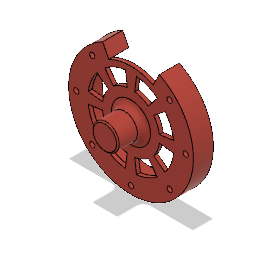
Hip Axis (Autodesk Fusion 360 design; units mm, degrees)
Autodesk Fusion 360 part; units mm, degrees
sketch "base" plane through (0, 0, 0) normal (0, 0, 1) x (1, 0, 0)
  circle A0 centre (0, 0) radius 48
  circle A1 centre (0, 0) radius 37.5
  line L0 (0, 0) -> (0, 48)
  line L1 (0, 0) -> (-21.7169, 42.8063)
  line L2 (0, 0) -> (21.7169, 42.8063)
  dimension "d1" = 96
  dimension "d2" = 75
  dimension "d3" = 26.9
  constraint coincident A0.centre A1.centre
  constraint concentric A0 A1
  constraint coincident A0 L0.end
  constraint vertical L0
  constraint coincident A0 L1.end
  constraint symmetric L0 A0.centre A1.centre
  constraint symmetric L0 L1.end L2.end
  measures "d1" diameter of A0
  measures "d2" diameter of A1
  measures "d3" angle of L0 L1
extrude "Extrude1" add sketch "base" against normal blind 15.5 contours A0 A1 L1 L2
extrude "Extrude2" add sketch "base" against normal blind 3 contours A1 L0 L2 | A1 L1 L2 | A1 L0 L1
sketch "axis" plane through (0, 0, 0) normal (0, 0, 1) x (1, 0, 0)
  circle A0 centre (0, 0) radius 10
  dimension "d8" = 20
  constraint coincident A0.centre origin
  measures "d8" diameter of A0
extrude "Extrude3" add sketch "axis" along normal blind 20
fillet "Fillet1" radius 5 1 edges at (-9.3233, 3.6162, 0)
fillet "Fillet2" radius 1 1 edges at (-9.3233, -3.6162, 20)
sketch "thermal gaps" plane through (0, 0, 0) normal (0, 0, 1) x (1, 0, 0)
  line L0 (0, 0) -> (0, -65)
  line L1 (0, 0) -> (4.3074, -32.7177)
  line L2 (0, 0) -> (2.8716, -21.8118)
  line L3 (0, 0) -> (13.3928, -17.4538)
  line L4 (0, 0) -> (20.0891, -26.1807)
  arc A0 (2.8716, -21.8118) -> (13.3928, -17.4538) centre (0, 0) ccw
  arc A1 (4.3074, -32.7177) -> (20.0891, -26.1807) centre (0, 0) ccw
  line L5 (20.0891, -26.1807) -> (13.3928, -17.4538)
  line L6 (4.3074, -32.7177) -> (2.8716, -21.8118)
  line L7 (32.7177, -4.3074) -> (21.8118, -2.8716)
  line L8 (26.1807, -20.0891) -> (17.4538, -13.3928)
  arc A2 (17.4538, -13.3928) -> (21.8118, -2.8716) centre (0, 0) ccw
  arc A3 (26.1807, -20.0891) -> (32.7177, -4.3074) centre (0, 0) ccw
  line L9 (26.1807, 20.0891) -> (17.4538, 13.3928)
  line L10 (32.7177, 4.3074) -> (21.8118, 2.8716)
  arc A4 (21.8118, 2.8716) -> (17.4538, 13.3928) centre (0, 0) ccw
  arc A5 (32.7177, 4.3074) -> (26.1807, 20.0891) centre (0, 0) ccw
  line L11 (4.3074, 32.7177) -> (2.8716, 21.8118)
  line L12 (20.0891, 26.1807) -> (13.3928, 17.4538)
  arc A6 (13.3928, 17.4538) -> (2.8716, 21.8118) centre (0, 0) ccw
  arc A7 (20.0891, 26.1807) -> (4.3074, 32.7177) centre (0, 0) ccw
  line L13 (-20.0891, 26.1807) -> (-13.3928, 17.4538)
  line L14 (-4.3074, 32.7177) -> (-2.8716, 21.8118)
  arc A8 (-2.8716, 21.8118) -> (-13.3928, 17.4538) centre (0, 0) ccw
  arc A9 (-4.3074, 32.7177) -> (-20.0891, 26.1807) centre (0, 0) ccw
  line L15 (-32.7177, 4.3074) -> (-21.8118, 2.8716)
  line L16 (-26.1807, 20.0891) -> (-17.4538, 13.3928)
  arc A10 (-17.4538, 13.3928) -> (-21.8118, 2.8716) centre (0, 0) ccw
  arc A11 (-26.1807, 20.0891) -> (-32.7177, 4.3074) centre (0, 0) ccw
  line L17 (-26.1807, -20.0891) -> (-17.4538, -13.3928)
  line L18 (-32.7177, -4.3074) -> (-21.8118, -2.8716)
  arc A12 (-21.8118, -2.8716) -> (-17.4538, -13.3928) centre (0, 0) ccw
  arc A13 (-32.7177, -4.3074) -> (-26.1807, -20.0891) centre (0, 0) ccw
  line L19 (-4.3074, -32.7177) -> (-2.8716, -21.8118)
  line L20 (-20.0891, -26.1807) -> (-13.3928, -17.4538)
  arc A14 (-13.3928, -17.4538) -> (-2.8716, -21.8118) centre (0, 0) ccw
  arc A15 (-20.0891, -26.1807) -> (-4.3074, -32.7177) centre (0, 0) ccw
  dimension "d15" = 33
  dimension "d16" = 7.5
  dimension "d17" = 22
  dimension "d18" = 22
  dimension "d19" = 33
  dimension "d20" = 30
  dimension "d22" = 360
  constraint coincident L0.start L1.start
  constraint vertical L0
  constraint parallel L1 L2
  constraint parallel L3 L4
  measures "d15" distance of L0.start L1.end
  measures "d16" angle of L0.start L0.end L1.end
  measures "d17" distance of L0.start L2.end
  measures "d18" distance of L0.start L3.end
  measures "d19" distance of L0.start L4.end
  measures "d20" angle of L0.start L2.end L3.end
extrude "Extrude4" cut sketch "thermal gaps" against normal blind 10 contours L1 L4 A0 A1 L5 L6 | L7 L8 A2 A3 | L9 L10 A4 A5 | L11 L12 A6 A7 | L13 L14 A8 A9 | L15 L16 A10 A11 | L17 L18 A12 A13 | L19 L20 A14 A15
sketch "Sketch5" plane through (0, 0, 0) normal (0, 0, 1) x (1, 0, 0)
  line L0 (0, 0) -> (0, 42)
  circle A0 centre (0, 42) radius 2
  circle A1 centre (-29.6985, 29.6985) radius 2
  circle A2 centre (-42, 0) radius 2
  circle A3 centre (-29.6985, -29.6985) radius 2
  circle A4 centre (0, -42) radius 2
  circle A5 centre (29.6985, -29.6985) radius 2
  circle A6 centre (42, 0) radius 2
  circle A7 centre (29.6985, 29.6985) radius 2
  dimension "d25" = 42
  dimension "d26" = 4
  dimension "d28" = 360
  constraint coincident L0.start origin
  constraint vertical L0
  constraint coincident L0.end A0.centre
  measures "d25" distance of L0.start L0.end
  measures "d26" diameter of A0
extrude "Extrude5" cut sketch "Sketch5" against normal blind 25 contours A1 | A2 | A3 | A4 | A5 | A6 | A7
equation "d3 = ( 53.8 / 2 ) * 1 deg"
named bodies: "base"
